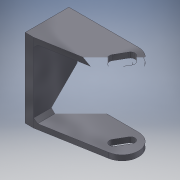
# Autodesk Inventor part: Solder Roll Support 2
Saved by Autodesk Inventor 2016 (Build 200138000, 138)
## iProperties
Created: 2017-09-04
Part Number: Solder Roll Support 2
Material: SAE 1020
Document SubType Name: Modeling
Designer: Zigunov
Stock Number: 0
Mass: 1729.01 g
Surface Area: 745.421 cm^2
Volume: 219.697 cm^3
Density: 7.87 g/cm^3
Appearance: Steel - Polished
Author: Zigunov
Autodesk Inventor part; units mm, degrees
ref_plane "YZ Plane" through (0, 0, 0) normal (1, 0, 0) x (0, 1, 0)
ref_plane "XZ Plane" through (0, 0, 0) normal (0, 1, 0) x (-1, 0, 0)
ref_plane "XY Plane" through (0, 0, 0) normal (0, 0, 1) x (1, 0, 0)
sketch "Sketch2" plane through (0, 0, 0) normal (0, 0, 1) x (1, 0, 0)
  line L0 (0, 0) -> (4.8, 0)
  line L1 (4.8, 0) -> (4.8, 25)
  line L2 (4.8, 25) -> (0, 25)
  line L3 (0, 25) -> (0, 0)
  dimension "d11" = 25
  dimension "d12" = 4.8
  constraints: 8 end point, 2 parallel, 1 horizontal, 1 perpendicular
  measures "d11" distance of L2.end L0.start
  measures "d12" distance of L1.end L2.end
extrude "Extrusion2" add sketch "Sketch2" along normal mid plane 45
sketch "Sketch3" plane through (0, 0, 22.5) normal (0, 0, 1) x (1, 0, 0)
  line L0 (4.8, 0) -> (4.8, 25) projected
  line L1 (4.8, 25) -> (44.8, 25)
  line L2 (44.8, 25) -> (45.7352, 3.5814) construction
  line L3 (45.7352, 3.5814) -> (4.8, 0)
  arc A0 (45.7352, 3.5814) -> (44.8, 25) centre (44.8, 14.2703) ccw
  line L4 (46.55, 17.3014) -> (43.05, 11.2392) construction
  line L5 (44.3849, 18.5514) -> (40.8849, 12.4892)
  line L6 (45.2151, 9.9892) -> (48.7151, 16.0514)
  arc A1 (48.7151, 16.0514) -> (44.3849, 18.5514) centre (46.55, 17.3014) ccw
  arc A2 (40.8849, 12.4892) -> (45.2151, 9.9892) centre (43.05, 11.2392) ccw
  point P0 (0, 0)
  dimension "d15" = 40
  dimension "d16" = 85
  dimension "d17" = 5
  dimension "d18" = 7
  dimension "d19" = 30
  constraints: 14 end point, 6 point on circle, 6 tangent, 3 centre point, 1 coincident, 1 midpoint, 1 parallel, 1 perpendicular
  measures "d15" distance from line of L0 point (44.8, 14.27)
  measures "d16" angle of L0 L3
  measures "d17" distance between parallel lines of L5 L6
  measures "d18" distance of L4.start L4.end
  measures "d19" angle of L0 L4
extrude "Extrusion3" add sketch "Sketch3" against normal blind 3
mirror "Mirror1" about plane through (0, 0, 0) normal (0, 0, 1) of "Extrusion3"
chamfer "Chamfer1" distance 2 angle 45 2 edges at (4.8, 12.5, 19.5) (4.8, 12.5, -19.5)
body "Solid2"
